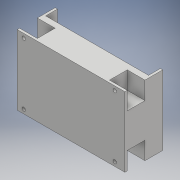
# Autodesk Inventor part: ultra96_holder
Saved by Autodesk Inventor 2018 (Build 220112000, 112)
## iProperties
Created: 2019-07-22
Part Number: ultra96_holder
Material: 一般
Document SubType Name: Modeling
Designer: guest1
Density: 1 g/cm^3
Appearance: 既定
Author: guest1
Autodesk Inventor part; units mm, degrees
ref_plane "YZ Plane" through (0, 0, 0) normal (1, 0, 0) x (0, 1, 0)
ref_plane "XZ Plane" through (0, 0, 0) normal (0, 1, 0) x (-1, 0, 0)
ref_plane "XY Plane" through (0, 0, 0) normal (0, 0, 1) x (1, 0, 0)
sketch "スケッチ1" plane through (0, 0, 0) normal (0, 0, 1) x (1, 0, 0)
  line L0 (-45.5, -42) -> (45.5, -42)
  line L1 (45.5, -42) -> (45.5, 22)
  line L2 (45.5, 22) -> (-45.5, 22)
  line L3 (-45.5, 22) -> (-45.5, -42)
  line L4 (-45.5, 0) -> (0, 0)
  line L5 (0, 0) -> (45.5, 0)
  dimension "d0" = 64
  dimension "d1" = 91
  dimension "d20" = 42
  constraints: 12 end point, 3 point on line, 2 horizontal, 2 parallel, 1 collinear, 1 perpendicular
  measures "d0" distance of L2.end L0.start
  measures "d1" distance of L1.end L2.end
  measures "d20" distance from line of L0 L4.end
extrude "外枠2" add sketch "スケッチ1" along normal blind 59
sketch "スケッチ２" plane through (0, 0, 0) normal (0, 0, -1) x (1, 0, 0)
  line L0 (43.5, -20) -> (-43.5, -20)
  line L1 (-43.5, -20) -> (-43.5, 20)
  line L2 (-43.5, 20) -> (43.5, 20)
  line L3 (43.5, 20) -> (43.5, -20)
  line L4 (43.5, -20) -> (-43.5, 20) construction
  line L5 (-43.5, -20) -> (43.5, 20) construction
  point P0 (0, 0)
  dimension "d4" = 40
  dimension "d5" = 87
  constraints: 12 end point, 2 midpoint, 2 parallel, 1 horizontal, 1 perpendicular
  measures "d4" distance of L0.end L1.end
  measures "d5" distance of L1.end L2.end
extrude "本体" cut sketch "スケッチ２" against normal blind 59
sketch "スケッチ4" plane through (-45.5, 22, 0) normal (0, 1, 0) x (1, 0, 0)
  line L0 (0, -59) -> (91, -59) projected
  line L1 (0, 0) -> (91, 0) projected
  line L2 (91, -59) -> (0, -59)
  line L3 (0, -59) -> (0, 0)
  line L4 (0, 0) -> (91, 0)
  line L5 (91, 0) -> (91, -59)
  point P0 (45.5, 0)
  constraints: 8 end point, 2 parallel, 1 horizontal, 1 perpendicular
extrude "上くり抜き" cut sketch "スケッチ4" against normal blind 2
sketch "スケッチ5" plane through (0, 0, 0) normal (0, 0, -1) x (-1, 0, 0)
  line L0 (-43.5, -20) -> (-43.5, 20) projected
  line L1 (-43.5, 20) -> (-38.5, 20)
  line L2 (-38.5, 20) -> (-38.5, -13)
  line L3 (-38.5, -13) -> (33.5, -13)
  line L4 (33.5, -13) -> (33.5, 20)
  line L5 (43.5, -20) -> (43.5, 20) projected
  line L6 (33.5, 20) -> (43.5, 20)
  line L7 (43.5, 20) -> (43.5, -20)
  line L8 (43.5, -20) -> (-43.5, -20) projected
  line L9 (43.5, -20) -> (-43.5, -20)
  line L10 (-43.5, -20) -> (-43.5, 20)
  point P0 (0, 0)
  dimension "d15" = 5
  dimension "d16" = 10
  dimension "d17" = 33
  constraints: 16 end point, 4 perpendicular, 2 collinear, 2 horizontal, 1 point on line
  measures "d15" distance of L0.end L1.end
  measures "d16" distance of L4.end L5.end
  measures "d17" distance of L1.end L2.end
extrude "側面" add sketch "スケッチ5" against normal blind 2
sketch "スケッチ6" plane through (43.5, -20, 59) normal (-1, 0, 0) x (0, 0, 1)
  line L0 (-49, 5.5) -> (-29, 5.5)
  line L1 (-29, 5.5) -> (-29, 1.5)
  line L2 (-29, 1.5) -> (-49, 1.5)
  line L3 (-49, 1.5) -> (-49, 5.5)
  line L4 (-17, 5.5) -> (-7, 5.5)
  line L5 (-7, 5.5) -> (-7, 1.5)
  line L6 (-7, 1.5) -> (-17, 1.5)
  line L7 (-17, 1.5) -> (-17, 5.5)
  line L8 (-57, 0) -> (0, 0) projected
  line L9 (0, 40) -> (0, 0) projected
  point P0 (-59, 20)
  point P1 (-57, 7)
  dimension "d21" = 1.5
  dimension "d22" = 8
  dimension "d23" = 20
  dimension "d24" = 10
  dimension "d25" = 7
  dimension "d26" = 4
  dimension "d27" = 4
  constraints: 16 end point, 4 parallel, 2 horizontal, 2 perpendicular, 1 point on line
  measures "d21" distance between parallel lines of L8 L2
  measures "d22" distance from line of point (-57, 7) L3
  measures "d23" distance of L0.start L0.end
  measures "d24" distance of L4.start L4.end
  measures "d25" distance between parallel lines of L9 L5
  measures "d26" distance of L0.end L1.end
  measures "d27" distance of L4.end L5.end
extrude "支え" add sketch "スケッチ6" along normal blind 15
sketch "スケッチ9" plane through (0, 0, 0) normal (0, 0, -1) x (-1, 0, 0)
  line L0 (-45.5, -42) -> (-45.5, 20) projected
  line L1 (-45.5, -25) -> (-30.5, -25)
  line L2 (-30.5, -25) -> (-30.5, -40)
  line L3 (-30.5, -40) -> (-45.5, -40)
  line L4 (-45.5, -40) -> (-45.5, -25)
  line L5 (45.5, 20) -> (45.5, -42) projected
  line L6 (45.5, -25) -> (30.5, -25)
  line L7 (30.5, -25) -> (30.5, -40)
  line L8 (30.5, -40) -> (45.5, -40)
  line L9 (45.5, -40) -> (45.5, -25)
  line L10 (45.5, -42) -> (-45.5, -42) projected
  point P0 (0, 0)
  dimension "d38" = 2
  dimension "d39" = 15
  dimension "d40" = 15
  dimension "d41" = 15
  constraints: 16 end point, 4 parallel, 4 point on line, 2 horizontal, 2 perpendicular
  measures "d38" distance between parallel lines of L10 L3
  measures "d39" distance of L1.end L2.end
  measures "d40" distance of L2.end L3.end
  measures "d41" distance of L7.end L8.end
extrude "ネジ穴1" cut sketch "スケッチ9" against normal blind 15
sketch "スケッチ10" plane through (0, 0, 59) normal (0, 0, 1) x (1, 0, 0)
  line L0 (-45.5, -25) -> (-45.5, -40) projected
  line L1 (-45.5, -25) -> (-30.5, -25)
  line L2 (-30.5, -25) -> (-30.5, -40)
  line L3 (-30.5, -40) -> (-45.5, -40)
  line L4 (-45.5, -40) -> (-45.5, -25)
  line L5 (45.5, -40) -> (45.5, -25) projected
  line L6 (45.5, -25) -> (30.5, -25)
  line L7 (30.5, -25) -> (30.5, -40)
  line L8 (30.5, -40) -> (45.5, -40)
  line L9 (45.5, -40) -> (45.5, -25)
  line L10 (-45.5, -42) -> (45.5, -42) projected
  point P0 (0, 0)
  dimension "d44" = 15
  dimension "d45" = 2
  dimension "d46" = 2
  dimension "d47" = 15
  dimension "d48" = 15
  dimension "d49" = 15
  constraints: 16 end point, 4 parallel, 2 horizontal, 2 perpendicular, 2 point on line
  measures "d44" distance of L1.start L1.end
  measures "d45" distance between parallel lines of L10 L3
  measures "d46" distance between parallel lines of L10 L8
  measures "d47" distance of L1.end L2.end
  measures "d48" distance of L6.start L6.end
  measures "d49" distance of L6.end L7.end
extrude "ネジ穴2" cut sketch "スケッチ10" against normal blind 15
sketch "スケッチ15" plane through (-45.5, 20, 0) normal (0, 1, 0) x (1, 0, 0)
  line L0 (76, -59) -> (91, -59) projected
  line L1 (84, 0) -> (91, 0) projected
  line L2 (91, -59) -> (91, 0)
  line L3 (91, 0) -> (84, 0)
  line L4 (84, 0) -> (84, -2) projected
  line L5 (84, 0) -> (84, -2)
  line L6 (89, -2) -> (84, -2) projected
  line L7 (84, -2) -> (89, -2)
  line L8 (89, -2) -> (89, -59) projected
  line L9 (89, -2) -> (89, -59)
  line L10 (89, -59) -> (2, -59) projected
  line L11 (2, -2) -> (2, -59) projected
  line L12 (2, -59) -> (2, -2)
  line L13 (84, -2) -> (12, -2) projected
  line L14 (2, -2) -> (12, -2)
  line L15 (12, 0) -> (12, -2) projected
  line L16 (12, -2) -> (12, 0)
  line L17 (15, 0) -> (0, 0) projected
  line L18 (12, 0) -> (0, 0)
  line L19 (0, 0) -> (0, -59) projected
  line L20 (0, 0) -> (0, -59)
  line L21 (0, -59) -> (2, -59)
  point P0 (45.5, 0)
  constraints: 22 end point, 6 perpendicular, 4 collinear, 1 parallel
extrude "押し出し11" cut sketch "スケッチ15" against normal blind 30 contours L8 L6 L4 L1 L2 L0 | L21 L19 L17 L15 L14 L11
sketch "スケッチ17" plane through (-45.5, -42, 0) normal (0, -1, 0) x (1, 0, 0)
  line L0 (91, 59) -> (91, 44) projected
  line L1 (15, 0) -> (0, 0) projected
  line L2 (91, 0) -> (91, 59) projected
  line L3 (5.5, 3.5) -> (82.5, 3.5)
  line L4 (82.5, 3.5) -> (82.5, 55.5)
  line L5 (82.5, 55.5) -> (5.5, 55.5)
  line L6 (5.5, 55.5) -> (5.5, 3.5)
  line L7 (5.5, 3.5) -> (82.5, 55.5) construction
  line L8 (82.5, 3.5) -> (5.5, 55.5) construction
  point P0 (45.5, 0)
  point P1 (44, 29.5)
  dimension "d55" = 77
  dimension "d56" = 52
  constraints: 12 end point, 2 midpoint, 2 parallel, 1 horizontal, 1 perpendicular
  measures "d55" distance of L4.end L5.end
  measures "d56" distance of L3.end L4.end
hole "穴1" at (-40, -42, 55.5) at (-40, -42, 3.5) at (37, -42, 55.5) at (37, -42, 3.5) direction (0, 1, 0) diameter 3 depth 2 tip angle 118
